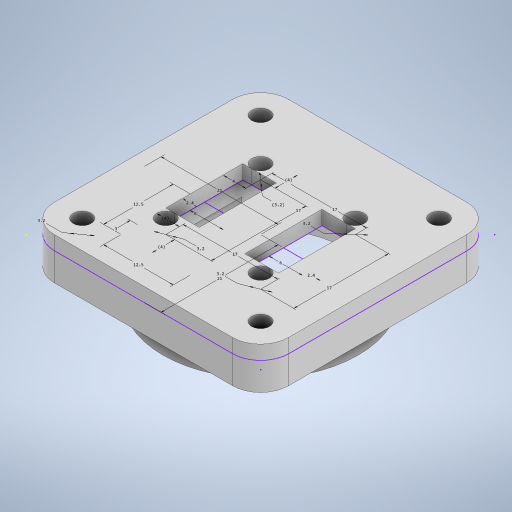
# Autodesk Inventor part: mounter
Saved by Autodesk Inventor 2024 (Build 280153000, 153)
## iProperties
Created: 2024-02-10
Part Number: mounter
Material: 一般
Document SubType Name: Modeling
Designer: mott1
Density: 1 g/cm^3
Appearance: 既定
Author: mott1
Autodesk Inventor part; units mm, degrees
ref_plane "YZ Plane" through (0, 0, 0) normal (1, 0, 0) x (0, 1, 0)
ref_plane "XZ Plane" through (0, 0, 0) normal (0, 1, 0) x (-1, 0, 0)
ref_plane "XY Plane" through (0, 0, 0) normal (0, 0, 1) x (1, 0, 0)
sketch "スケッチ1" plane through (0, 0, 0) normal (0, 1, 0) x (-1, 0, 0)
  line L0 (-5, 0) -> (-21, 0)
  line L1 (-21, -21) -> (0, -21)
  line L2 (0, -21) -> (0, -5)
  arc A0 (0, -5) -> (-5, 0) centre (-5, -5) ccw
  line L3 (0, -5) -> (0, -8)
  circle A1 centre (-5, -5) radius 1.6
  line L4 (-21, -21) -> (-8.5, -21)
  line L5 (-8.5, -21) -> (-8.5, -8.5)
  line L6 (-8.5, -8.5) -> (-21, -8.5)
  line L7 (-8.5, -8.5) -> (-8.5, -11.5)
  circle A2 centre (-12.5, -12.5) radius 1.6
  line L8 (-5, -42) -> (-21, -42)
  line L9 (0, -21) -> (0, -37)
  arc A3 (-5, -42) -> (0, -37) centre (-5, -37) ccw
  line L10 (0, -37) -> (0, -34)
  circle A4 centre (-5, -37) radius 1.6
  line L11 (-8.5, -21) -> (-8.5, -33.5)
  line L12 (-8.5, -33.5) -> (-21, -33.5)
  line L13 (-8.5, -33.5) -> (-8.5, -30.5)
  circle A5 centre (-12.5, -29.5) radius 1.6
  line L14 (-37, 0) -> (-21, 0)
  line L15 (-21, -21) -> (-42, -21)
  line L16 (-42, -21) -> (-42, -5)
  arc A6 (-37, 0) -> (-42, -5) centre (-37, -5) ccw
  line L17 (-42, -5) -> (-42, -8)
  circle A7 centre (-37, -5) radius 1.6
  line L18 (-21, -21) -> (-33.5, -21)
  line L19 (-33.5, -21) -> (-33.5, -8.5)
  line L20 (-33.5, -8.5) -> (-21, -8.5)
  line L21 (-33.5, -8.5) -> (-33.5, -11.5)
  circle A8 centre (-29.5, -12.5) radius 1.6
  circle A9 centre (-37, -37) radius 1.6
  line L22 (-42, -37) -> (-42, -34)
  line L23 (-33.5, -33.5) -> (-33.5, -30.5)
  circle A10 centre (-29.5, -29.5) radius 1.6
  line L24 (-37, -42) -> (-21, -42)
  line L25 (-42, -21) -> (-42, -37)
  line L26 (-33.5, -33.5) -> (-21, -33.5)
  line L27 (-33.5, -21) -> (-33.5, -33.5)
  arc A11 (-42, -37) -> (-37, -42) centre (-37, -37) ccw
  line L28 (-10.9, -14.1) -> (-16.9, -14.1)
  line L29 (-16.9, -14.1) -> (-16.9, -27.9)
  line L30 (-16.9, -27.9) -> (-10.9, -27.9)
  line L31 (-10.9, -27.9) -> (-10.9, -14.1)
  line L32 (-31.1, -14.1) -> (-25.1, -14.1)
  line L33 (-25.1, -14.1) -> (-25.1, -27.9)
  line L34 (-25.1, -27.9) -> (-31.1, -27.9)
  line L35 (-31.1, -27.9) -> (-31.1, -14.1)
  point P0 (0, 0)
  point P1 (0, -42)
  point P2 (-42, 0)
  point P3 (-42, -42)
  point P4 (-12.5, -14.1)
  point P5 (-12.5, -27.9)
  point P6 (-29.5, -14.1)
  point P7 (-29.5, -27.9)
  dimension "d0" = 21
  dimension "d1" = 21
  dimension "d6" = 3.2
  dimension "d7" = 12.5
  dimension "d8" = 12.5
  dimension "d9" = 3
  dimension "d11" = 3.2
  dimension "d21" = 17
  dimension "d22" = 17
  dimension "d23" = 17
  dimension "d24" = 17
  dimension "d25" = 4
  dimension "d26" = 4
  dimension "d27" = 4
  dimension "d28" = 4
  dimension "d29" = 3.2
  dimension "d30" = 3.2
  dimension "d31" = 3.2
  dimension "d32" = 2.4
  dimension "d33" = 2.4
  dimension "d34" = 6
  dimension "d35" = 6
  constraints: 72 end point, 12 centre point, 11 symmetric about line, 8 point on circle, 8 point on line, 6 parallel, 4 coincident, 4 horizontal, 3 perpendicular, 3 other
  measures "d0" distance of L1.end L1.start
  measures "d1" distance of L1.start L0.end
  measures "d6" diameter of A1
  measures "d7" distance of L6.end L5.end
  measures "d8" distance of L5.end L4.end
  measures "d9" distance of L5.end L7.end
  measures "d11" diameter of A2
  measures "d21" distance of A8.centre A2.centre
  measures "d22" distance of A5.centre A2.centre
  measures "d23" distance of A8.centre A10.centre
  measures "d24" distance of A5.centre A10.centre
  measures "d25" distance from line of L6 A2.centre
  measures "d26" distance from line of L12 A5.centre
  measures "d27" distance from line of L11 A5.centre
  measures "d28" distance from line of L5 A2.centre
  measures "d29" diameter of A5
  measures "d30" diameter of A10
  measures "d31" diameter of A8
  measures "d32" distance between parallel lines of L5 L31
  measures "d33" distance between parallel lines of L35 L19
  measures "d34" distance between parallel lines of L33 L35
  measures "d35" distance between parallel lines of L31 L29
extrude "押し出し2" add sketch "スケッチ1" against normal blind 5 contours A0 L2 L1 L5 L6 L20 L19 L15 L16 A6 L14 L0 | L9 A3 L8 L24 A11 L22 L25 L15 L27 L23 L26 L12 L11 L1
sketch "スケッチ2" plane through (0, -5, 0) normal (0, -1, 0) x (1, 0, 0)
  line L0 (33.5, -8.5) -> (8.5, -8.5) projected
  line L1 (8.5, -33.5) -> (33.5, -33.5) projected
  line L2 (33.5, -8.5) -> (8.5, -8.5)
  line L3 (8.5, -8.5) -> (8.5, -33.5)
  line L4 (8.5, -33.5) -> (33.5, -33.5)
  line L5 (33.5, -33.5) -> (33.5, -8.5)
  arc A0 (8.5, -8.7526) -> (8.5, -33.2473) centre (21.0001, -21) ccw
  arc A1 (8.5, -11.8349) -> (8.5, -30.165) centre (21.0001, -21) ccw
  arc A2 (30.1653, -8.5) -> (11.8349, -8.5) centre (21.0001, -21) ccw
  arc A3 (33.2476, -8.5) -> (8.7526, -8.5) centre (21.0001, -21) ccw
  arc A4 (11.835, -33.5) -> (30.1652, -33.5) centre (21.0001, -21) ccw
  arc A5 (33.5, -30.1652) -> (33.5, -11.8347) centre (21.0001, -21) ccw
  arc A6 (8.7527, -33.5) -> (33.2475, -33.5) centre (21.0001, -21) ccw
  arc A7 (33.5, -33.2475) -> (33.5, -8.7524) centre (21.0001, -21) ccw
  point P0 (0, 0)
  point P1 (30.1652, -33.5)
  point P2 (33.2476, -8.5)
  point P3 (8.7526, -8.5)
  point P4 (11.8349, -8.5)
  constraints: 16 point on circle, 16 point on line, 8 centre point, 8 end point, 2 parallel, 1 coincident, 1 horizontal, 1 perpendicular
extrude "押し出し3" add sketch "スケッチ2" along normal blind 5 contours L0 A2 A3 | A7 L5 A5 | L3 A1 A0 | A6 L1 A4
extrude "押し出し4" add sketch "スケッチ1" along normal blind 2.5 contours A0 L2 L1 L5 L6 L20 L19 L15 L16 A6 L14 L0 | L9 A3 L8 L24 A11 L22 L25 L15 L27 L23 L26 L12 L11 L1 | L11 L12 L26 L23 L27 L15 L35 L34 L33 L1 L29 L30 L31 | L1 L31 L28 L29 L15 L33 L32 L35 L19 L20 L6 L5
